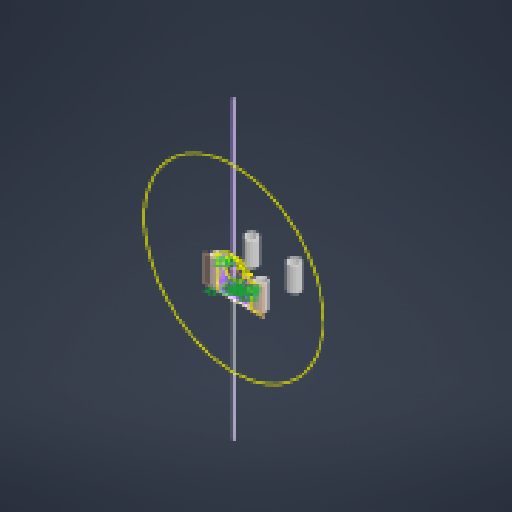
# Autodesk Inventor part: FastenerForLegFrame
Saved by Autodesk Inventor 2027 (Build 310192000, 192)
## iProperties
Created: 2026-07-09
Part Number: FastenerForLegFrame
Material: Generic
Document SubType Name: Modeling
Designer: belcz
Density: 1 g/cm^3
Appearance: Default
Author: belcz
Autodesk Inventor part; units mm, degrees
ref_plane "YZ Plane" through (0, 0, 0) normal (1, 0, 0) x (0, 1, 0)
ref_plane "XZ Plane" through (0, 0, 0) normal (0, 1, 0) x (-1, 0, 0)
ref_plane "XY Plane" through (0, 0, 0) normal (0, 0, 1) x (1, 0, 0)
sketch "Sketch1" plane through (0, 0, 0) normal (0, 1, 0) x (-1, 0, 0)
  arc A0 (17.7231, -22.7881) -> (17.7231, -20.9526) centre (20.7626, -21.8703) ccw projected
  arc A1 (17.7231, -20.9526) -> (17.7231, -22.7881) centre (20.7626, -21.8703) ccw projected
  arc A2 (17.7231, -48.6072) -> (17.7231, -46.7717) centre (20.7626, -47.6894) ccw projected
  arc A3 (17.7231, -46.7717) -> (17.7231, -48.6072) centre (20.7626, -47.6894) ccw projected
  arc A4 (-9.726, -46.7717) -> (-9.726, -48.6072) centre (-12.7654, -47.6894) ccw projected
  arc A5 (-9.726, -48.6072) -> (-9.726, -46.7717) centre (-12.7654, -47.6894) ccw projected
  arc A6 (-9.726, -20.9526) -> (-9.726, -22.7881) centre (-12.7654, -21.8703) ccw projected
  arc A7 (-9.726, -22.7881) -> (-9.726, -20.9526) centre (-12.7654, -21.8703) ccw projected
  circle A8 centre (20.7626, -21.8703) radius 3.429
  circle A9 centre (20.7626, -47.6894) radius 3.429
  circle A10 centre (-12.7654, -47.6894) radius 3.429
  circle A11 centre (-12.7654, -21.8703) radius 3.429
  circle A12 centre (-12.7654, -21.8703) radius 4.445
  circle A13 centre (-12.7654, -47.6894) radius 4.445
  circle A14 centre (20.7626, -47.6894) radius 4.445
  circle A15 centre (20.7626, -21.8703) radius 4.445
  point P0 (0, 0)
  dimension "d0" = 6.858
  dimension "d1" = 6.858
  dimension "d2" = 6.858
  dimension "d3" = 6.858
  dimension "d4" = 8.89
  dimension "d5" = 8.89
  dimension "d6" = 8.89
  dimension "d7" = 8.89
  constraints: 8 centre point, 8 coincident
  measures "d0" diameter of A8
  measures "d1" diameter of A9
  measures "d2" diameter of A10
  measures "d3" diameter of A11
  measures "d4" diameter of A12
  measures "d5" diameter of A13
  measures "d6" diameter of A14
  measures "d7" diameter of A15
extrude "Extrusion1" add sketch "Sketch1" along normal blind 19.05 contours A12 | A13 | A14 | A15
ref_plane "Work Plane2" through (-20.7626, 0, -17.4253) normal (0, 0, 1) x (1, 0, 0)
ref_plane "Work Plane1" through (-4.353, 20.3962, -73.6634) normal (0, 0, 1) x (1, 0, 0)
sketch "Sketch2" plane through (-20.7626, 0, -17.4253) normal (0, 0, 1) x (1, 0, 0)
  circle A0 centre (16.4095, 20.3962) radius 7.9375 projected
  line L0 (29.718, 19.05) -> (28.448, 19.05) projected
  line L1 (29.083, 0) -> (29.083, 19.05) projected
  line L2 (29.718, 19.05) -> (37.0078, 19.05) projected
  circle A1 centre (16.4095, 20.3962) radius 69.85 projected
  circle A2 centre (16.4095, 20.3962) radius 7.9375 projected
  line L3 (29.3635, 19.05) -> (28.0935, 19.05) projected
  line L4 (28.0935, 22.098) -> (28.0935, 19.05) projected
  line L5 (26.8235, 20.5954) -> (28.0935, 19.1092) projected
  line L6 (22.3384, 25.8441) -> (26.8235, 20.5954) projected
  arc A3 (22.3384, 25.8441) -> (21.3729, 26.289) centre (21.3729, 25.019) ccw projected
  line L7 (4.7255, 19.05) -> (3.4555, 19.05) projected
  line L8 (4.445, 0) -> (4.445, 19.05) projected
  line L9 (4.7255, 19.1092) -> (5.9955, 20.5954) projected
  arc A4 (12.3827, 29.337) -> (7.5552, 27.1123) centre (12.3827, 22.987) ccw projected
  line L10 (7.5552, 27.1123) -> (3.6505, 22.5429) projected
  arc A5 (2.685, 22.098) -> (3.6505, 22.5429) centre (2.685, 23.368) ccw projected
  line L11 (5.9955, 22.098) -> (2.685, 22.098) projected
  line L12 (5.9955, 20.5954) -> (5.9955, 22.098) projected
  line L13 (5.9955, 20.5954) -> (10.4807, 25.8441) projected
  arc A6 (11.4462, 26.289) -> (10.4807, 25.8441) centre (11.4462, 25.019) ccw projected
  line L14 (11.4462, 26.289) -> (21.3729, 26.289) projected
  arc A7 (22.3384, 25.8441) -> (21.3729, 26.289) centre (21.3729, 25.019) ccw projected
  line L15 (22.3384, 25.8441) -> (26.8235, 20.5954) projected
  line L16 (26.8235, 22.098) -> (26.8235, 20.5954) projected
  line L17 (30.1341, 22.098) -> (26.8235, 22.098) projected
  arc A8 (29.1686, 22.5429) -> (30.1341, 22.098) centre (30.1341, 23.368) ccw projected
  line L18 (29.1686, 22.5429) -> (25.2639, 27.1123) projected
  arc A9 (25.2639, 27.1123) -> (20.4364, 29.337) centre (20.4364, 22.987) ccw projected
  line L19 (12.3827, 29.337) -> (20.4364, 29.337) projected
  line L20 (4.445, 19.05) -> (8.255, 19.05)
  line L21 (16.4095, 12.4587) -> (16.4095, 8.6487)
  arc A10 (8.3294, 19.05) -> (24.4897, 19.05) centre (16.4095, 20.3962) ccw
  line L22 (8.255, 19.05) -> (8.3294, 19.05)
  line L23 (24.4897, 19.05) -> (29.494, 19.05)
  line L24 (29.494, 16.51) -> (26.4127, 16.51)
  line L25 (6.4064, 16.51) -> (4.445, 16.51)
  line L26 (21.3729, 10.8814) -> (29.083, 3.1713)
  line L27 (21.3729, 10.8814) -> (34.2329, 10.8814) construction
  line L28 (23.3424, 12.2047) -> (29.083, 6.4641)
  line L29 (23.3424, 12.2047) -> (31.4608, 12.2047) construction
  line L30 (29.083, 6.4641) -> (29.083, 3.1713)
  line L31 (28.829, 6.3589) -> (23.3263, 11.8616)
  arc A11 (21.7932, 10.8203) -> (23.3263, 11.8616) centre (16.4095, 20.3962) ccw
  line L32 (28.829, 3.7845) -> (28.829, 6.3589)
  line L33 (23.3263, 11.8616) -> (23.3263, 9.2872)
  line L34 (23.3263, 9.2872) -> (25.9007, 9.2872)
  line L35 (25.9007, 9.2872) -> (25.9007, 6.7128)
  line L36 (25.9007, 6.7128) -> (28.475, 6.7128)
  line L37 (28.475, 6.7128) -> (28.475, 4.1385)
  arc A12 (23.3424, 12.2047) -> (26.4127, 16.51) centre (16.4095, 20.3962) ccw
  arc A13 (23.3263, 12.1911) -> (23.3424, 12.2047) centre (16.4095, 20.3962) ccw
  line L38 (37.973, 0) -> (29.083, 0) projected
  line L39 (4.445, 0) -> (29.083, 0)
  line L40 (16.4095, -95.1738) -> (16.4095, 135.9662)
  line L41 (29.083, 2.54) -> (29.083, 0)
  line L42 (4.445, 2.54) -> (4.445, 0)
  line L43 (30.099, 19.05) -> (30.099, 0) projected
  line L44 (28.829, 2.286) -> (4.699, 2.286)
  line L45 (4.699, 2.286) -> (4.699, 0.254)
  line L46 (4.699, 0.254) -> (28.829, 0.254)
  line L47 (28.829, 0.254) -> (28.829, 2.286)
  line L48 (28.221, 4.3925) -> (28.221, 6.4588)
  line L49 (28.221, 6.4588) -> (26.1547, 6.4588)
  line L50 (23.0723, 9.5412) -> (23.0723, 11.6618)
  line L51 (25.6467, 9.0332) -> (23.5803, 9.0332)
  line L52 (25.6467, 6.9668) -> (25.6467, 9.0332)
  line L53 (28.475, 4.1385) -> (28.829, 3.7845)
  line L54 (26.1547, 6.4588) -> (28.221, 4.3925)
  line L55 (21.7932, 10.8203) -> (23.0723, 9.5412)
  line L56 (23.5803, 9.0332) -> (25.6467, 6.9668)
  line L57 (4.699, 0.254) -> (6.731, 2.286)
  line L58 (4.699, 0.254) -> (7.5727, 0.254) construction
  line L59 (6.731, 2.286) -> (6.731, 0.254)
  line L60 (6.731, 0.254) -> (8.763, 2.286)
  line L61 (8.763, 0.254) -> (8.763, 2.286)
  line L62 (8.763, 0.254) -> (10.795, 2.286)
  line L63 (10.795, 2.286) -> (10.795, 0.254)
  line L64 (10.795, 0.254) -> (12.827, 2.286)
  line L65 (12.827, 2.286) -> (12.827, 0.254)
  line L66 (12.827, 0.254) -> (14.859, 2.286)
  line L67 (14.859, 2.286) -> (14.859, 0.254)
  line L68 (14.859, 0.254) -> (16.4095, 2.286)
  line L69 (28.1201, 0.254) -> (26.0881, 2.286)
  line L70 (26.0881, 2.286) -> (26.0881, 0.254)
  line L71 (26.0881, 0.254) -> (24.0561, 2.286)
  line L72 (24.0561, 0.254) -> (24.0561, 2.286)
  line L73 (24.0561, 0.254) -> (22.0241, 2.286)
  line L74 (22.0241, 2.286) -> (22.0241, 0.254)
  line L75 (22.0241, 0.254) -> (19.9921, 2.286)
  line L76 (19.9921, 2.286) -> (19.9921, 0.254)
  line L77 (19.9921, 0.254) -> (17.9601, 2.286)
  line L78 (17.9601, 2.286) -> (17.9601, 0.254)
  line L79 (17.9601, 0.254) -> (16.4095, 2.286)
  line L80 (23.8021, 0.8672) -> (22.3833, 2.286)
  line L81 (21.7701, 2.286) -> (21.7701, 0.8672)
  line L82 (21.7701, 0.8672) -> (20.3513, 2.286)
  line L83 (19.7381, 2.286) -> (19.7381, 0.8672)
  line L84 (19.7381, 0.8672) -> (18.3193, 2.286)
  line L85 (17.7061, 2.286) -> (17.7061, 1.0056)
  line L86 (17.7061, 1.0056) -> (16.729, 2.286)
  line L87 (16.09, 2.286) -> (15.113, 1.0056)
  line L88 (15.113, 1.0056) -> (15.113, 2.286)
  line L89 (14.4998, 2.286) -> (13.081, 0.8672)
  line L90 (13.081, 0.8672) -> (13.081, 2.286)
  line L91 (12.4678, 2.286) -> (11.049, 0.8672)
  line L92 (11.049, 0.8672) -> (11.049, 2.286)
  line L93 (10.4358, 2.286) -> (9.017, 0.8672)
  line L94 (9.017, 0.8672) -> (9.017, 2.286)
  line L95 (8.4038, 2.286) -> (6.985, 0.8672)
  line L96 (6.985, 0.8672) -> (6.985, 2.286)
  line L97 (6.3718, 2.286) -> (4.699, 0.6132)
  line L98 (28.2997, 0.4336) -> (28.4793, 0.254)
  line L99 (23.8021, 2.286) -> (23.8021, 0.8672)
  line L100 (25.8341, 0.8672) -> (24.4153, 2.286)
  line L101 (25.8341, 2.286) -> (25.8341, 0.8672)
  line L102 (28.2997, 0.4336) -> (26.4473, 2.286)
  line L103 (11.4462, 10.8814) -> (3.7361, 3.1713)
  line L104 (11.4462, 10.8814) -> (-1.4138, 10.8814) construction
  line L105 (9.4767, 12.2047) -> (3.7361, 6.4641)
  line L106 (3.9901, 6.3589) -> (9.4928, 11.8616)
  arc A14 (9.4928, 11.8616) -> (11.0259, 10.8203) centre (16.4095, 20.3962) ccw
  line L107 (3.9901, 3.7845) -> (3.9901, 6.3589)
  line L108 (9.4928, 11.8616) -> (9.4928, 9.2872)
  line L109 (9.4928, 9.2872) -> (6.9184, 9.2872)
  line L110 (6.9184, 9.2872) -> (6.9184, 6.7128)
  line L111 (6.9184, 6.7128) -> (4.344, 6.7128)
  line L112 (4.344, 6.7128) -> (4.344, 4.1385)
  line L113 (4.598, 4.3925) -> (4.598, 6.4588)
  line L114 (4.598, 6.4588) -> (6.6644, 6.4588)
  line L115 (9.7468, 9.5412) -> (9.7468, 11.6618)
  line L116 (7.1724, 9.0332) -> (9.2388, 9.0332)
  line L117 (7.1724, 6.9668) -> (7.1724, 9.0332)
  line L118 (4.344, 4.1385) -> (3.9901, 3.7845)
  line L119 (6.6644, 6.4588) -> (4.598, 4.3925)
  line L120 (11.0259, 10.8203) -> (9.7468, 9.5412)
  line L121 (9.2388, 9.0332) -> (7.1724, 6.9668)
  arc A15 (6.4064, 16.51) -> (9.4767, 12.2047) centre (16.4095, 20.3962) ccw
  arc A16 (11.4462, 10.8814) -> (21.3729, 10.8814) centre (16.4095, 20.3962) ccw
  line L122 (15.113, 2.286) -> (15.113, 9.7433)
  line L123 (17.7061, 2.54) -> (17.7061, 9.7433)
  line L124 (16.6635, 2.794) -> (17.4521, 3.5825)
  line L125 (17.4521, 3.8365) -> (16.6635, 3.8365)
  line L126 (16.6635, 4.0905) -> (17.4521, 4.8791)
  line L127 (17.4521, 5.1331) -> (16.6635, 5.1331)
  line L128 (16.6635, 5.3871) -> (17.4521, 6.1756)
  line L129 (17.4521, 6.4296) -> (16.6635, 6.4296)
  line L130 (16.6635, 6.6836) -> (17.4521, 7.4721)
  line L131 (17.4521, 7.7261) -> (16.6635, 7.7261)
  line L132 (16.6635, 7.9801) -> (17.4521, 8.7687)
  line L133 (17.4521, 9.0227) -> (16.6635, 9.0227)
  line L134 (16.6635, 9.2767) -> (17.072, 9.6852)
  line L135 (16.6635, 2.54) -> (17.4521, 2.54)
  line L136 (17.4521, 9.7433) -> (17.4521, 2.54)
  line L137 (16.6635, 2.54) -> (16.6635, 135.9662)
  line L138 (16.6635, -95.1738) -> (16.6635, -49.4533)
  line L139 (17.7061, 2.54) -> (29.083, 2.54)
  line L140 (4.445, 2.54) -> (16.4095, 2.54)
  line L141 (16.6635, 2.54) -> (17.4521, 2.54)
  line L142 (16.6962, 9.6685) -> (16.6635, 9.6359)
  line L143 (16.6635, 8.7687) -> (17.0929, 8.7687)
  line L144 (17.0929, 8.7687) -> (16.6635, 8.3394)
  line L145 (17.0929, 7.4721) -> (16.6635, 7.0428)
  line L146 (16.6635, 6.1756) -> (17.0929, 6.1756)
  line L147 (17.0929, 6.1756) -> (16.6635, 5.7463)
  line L148 (16.6635, 4.8791) -> (17.0929, 4.8791)
  line L149 (16.6635, 3.5825) -> (17.0929, 3.5825)
  line L150 (17.0929, 3.5825) -> (16.6635, 3.1532)
  line L151 (17.0929, 4.8791) -> (16.6635, 4.4497)
  line L152 (16.6635, 7.4721) -> (17.0929, 7.4721)
  line L153 (15.113, 2.54) -> (15.113, 9.7433)
  line L154 (16.1555, 2.794) -> (15.367, 3.5825)
  line L155 (15.367, 3.8365) -> (16.1555, 3.8365)
  line L156 (16.1555, 4.0905) -> (15.367, 4.8791)
  line L157 (15.367, 5.1331) -> (16.1555, 5.1331)
  line L158 (16.1555, 5.3871) -> (15.367, 6.1756)
  line L159 (15.367, 6.4296) -> (16.1555, 6.4296)
  line L160 (16.1555, 6.6836) -> (15.367, 7.4721)
  line L161 (15.367, 7.7261) -> (16.1555, 7.7261)
  line L162 (16.1555, 7.9801) -> (15.367, 8.7687)
  line L163 (15.367, 9.0227) -> (16.1555, 9.0227)
  line L164 (16.1555, 9.2767) -> (15.747, 9.6852)
  line L165 (16.1555, 2.54) -> (15.367, 2.54)
  line L166 (15.367, 9.7433) -> (15.367, 2.54)
  line L167 (16.1555, 2.54) -> (16.1555, 135.9662)
  line L168 (16.1555, 8.7687) -> (15.7262, 8.7687)
  line L169 (15.7262, 8.7687) -> (16.1555, 8.3394)
  line L170 (15.7262, 7.4721) -> (16.1555, 7.0428)
  line L171 (16.1555, 6.1756) -> (15.7262, 6.1756)
  line L172 (15.7262, 6.1756) -> (16.1555, 5.7463)
  line L173 (16.1555, 4.8791) -> (15.7262, 4.8791)
  line L174 (16.1555, 3.5825) -> (15.7262, 3.5825)
  line L175 (15.7262, 3.5825) -> (16.1555, 3.1532)
  line L176 (15.7262, 4.8791) -> (16.1555, 4.4497)
  line L177 (16.1555, 7.4721) -> (15.7262, 7.4721)
  line L178 (21.7932, 10.8203) -> (28.829, 3.7845)
  arc A17 (21.3729, 10.8814) -> (23.3263, 12.1911) centre (16.4095, 20.3962) ccw
  arc A18 (9.4767, 12.2047) -> (11.4462, 10.8814) centre (16.4095, 20.3962) ccw
  line L179 (3.7361, 6.4641) -> (3.7361, 3.1713)
  line L180 (3.7361, 3.1713) -> (3.7361, 6.4641)
  line L181 (3.7361, 6.4641) -> (3.7361, 3.1713)
  line L182 (16.4086, 29.337) -> (16.4086, -46.863)
  point P0 (20.7626, 0)
  dimension "d10" = 3.81
  dimension "d11" = 3.81
  dimension "d12" = 0.254
  dimension "d14" = 45
  dimension "d15" = 45
  dimension "d16" = 0.254
  dimension "d20" = 0.254
  dimension "d21" = 45
  dimension "d23" = 0.254
  dimension "d26" = 8.0538
  dimension "d27" = 76.2
  dimension "d28" = 4.0259
  constraints: 312 end point, 75 symmetric about line, 24 point on circle, 23 parallel, 21 point on line, 20 perpendicular, 9 centre point, 8 vertical, 5 horizontal, 2 collinear, 2 equal length, 1 vertical alignment, 114 other
  measures "d10" distance of L8.end L20.end
  measures "d11" distance of L21.start L21.end
  measures "d12" radial gap between concentric circles of A0 A10
  measures "d14" angle of L26 L27
  measures "d15" angle of L28 L29
  measures "d16" distance between parallel lines of L28 L31
  measures "d20" distance between parallel lines of L36 L49
  measures "d21" angle of L58 L57
  measures "d26" distance of L19.start L19.end
  measures "d27" distance of L182.start L182.end
  measures "d28" distance from line of L19.start L182
body "Solid1"
